Autodesk Fusion 360 part; units mm, degrees
(part 4 of 6)
  line L2387 (33.796111, 261.14375) -> (33.866667, 261.14375)
  line L2388 (10.442222, 231.61625) -> (10.089444, 231.475139)
  line L2389 (7.796389, 232.180694) -> (8.043333, 231.93375)
  line L2390 (28.998333, 231.651528) -> (29.068889, 231.722083)
  line L2391 (29.068889, 231.722083) -> (29.068889, 231.792639)
  line L2392 (28.292778, 227.347639) -> (28.222222, 227.312361)
  line L2393 (28.222222, 227.312361) -> (28.186944, 227.277083)
  line L2394 (28.186944, 227.277083) -> (28.151667, 227.17125)
  line L2395 (9.419167, 223.467083) -> (9.419167, 227.030139)
  line L2396 (16.086667, 223.220139) -> (16.016111, 223.149583)
  line L2397 (23.600833, 231.051805) -> (23.706667, 231.016528)
  line L2398 (23.495, 231.228194) -> (23.495, 231.157639)
  line L2399 (23.212778, 288.025417) -> (23.248056, 287.954861)
  line L2400 (23.248056, 287.954861) -> (23.212778, 287.81375)
  line L2401 (23.212778, 287.81375) -> (23.1775, 287.778472)
  line L2402 (5.961944, 223.184861) -> (6.067778, 223.114305)
  line L2403 (27.305, 252.88875) -> (27.340278, 252.641805)
  line L2404 (35.454167, 262.378472) -> (34.360556, 262.378472)
  line L2405 (41.521944, 265.377083) -> (41.768889, 265.341805)
  line L2406 (34.395833, 287.990139) -> (34.536944, 287.919583)
  line L2407 (35.806944, 289.648194) -> (35.806944, 289.507083)
  line L2408 (13.229167, 227.030139) -> (13.264444, 227.17125)
  line L2409 (36.83, 227.382917) -> (39.0525, 227.382917)
  line L2410 (43.991389, 288.836805) -> (43.991389, 287.390417)
  line L2411 (31.291389, 257.01625) -> (31.538333, 257.157361)
  line L2412 (31.538333, 257.157361) -> (31.785278, 257.369028)
  line L2413 (31.785278, 257.369028) -> (31.996944, 257.615972)
  line L2414 (31.996944, 257.615972) -> (32.138056, 257.898194)
  line L2415 (42.721389, 272.503194) -> (42.721389, 272.57375)
  line L2416 (42.721389, 272.57375) -> (42.686111, 272.644305)
  line L2417 (42.474444, 272.25625) -> (42.580278, 272.25625)
  line L2418 (8.396111, 226.85375) -> (8.501944, 226.85375)
  line L2419 (8.501944, 226.85375) -> (8.643056, 226.889028)
  line L2420 (8.643056, 226.889028) -> (8.678333, 226.924305)
  line L2421 (39.087778, 276.771805) -> (39.017222, 276.807083)
  line L2422 (39.193611, 276.277917) -> (39.228889, 276.419028)
  line L2423 (23.918333, 229.993472) -> (23.988889, 229.640694)
  line L2424 (17.78, 290.283194) -> (17.603611, 290.459583)
  line L2425 (13.440833, 223.114305) -> (13.335, 223.184861)
  line L2426 (14.781389, 280.722917) -> (14.499167, 280.687639)
  line L2427 (14.499167, 280.687639) -> (14.181667, 280.581805)
  line L2428 (14.181667, 280.581805) -> (13.899444, 280.440694)
  line L2429 (13.899444, 280.440694) -> (13.6525, 280.264305)
  line L2430 (39.299444, 265.659305) -> (39.405278, 265.624028)
  line L2431 (9.666111, 223.114305) -> (9.807222, 223.184861)
  line L2432 (9.807222, 223.184861) -> (9.877778, 223.220139)
  line L2433 (9.877778, 223.220139) -> (9.913056, 223.255417)
  line L2434 (26.387778, 253.20625) -> (26.916944, 253.20625)
  line L2435 (9.383889, 231.369305) -> (9.736667, 231.404583)
  line L2436 (15.769167, 223.114305) -> (13.581944, 223.114305)
  line L2437 (22.895278, 225.548472) -> (22.754167, 225.548472)
  line L2438 (23.106944, 224.172639) -> (23.106944, 225.195694)
  line L2439 (22.965833, 223.643472) -> (23.106944, 223.925694)
  line L2440 (23.106944, 223.925694) -> (23.106944, 224.172639)
  line L2441 (32.208611, 227.135972) -> (32.208611, 227.206528)
  line L2442 (32.208611, 227.206528) -> (32.138056, 227.277083)
  line L2443 (32.138056, 227.277083) -> (32.102778, 227.347639)
  line L2444 (40.181389, 240.329861) -> (40.287222, 240.400417)
  line L2445 (40.287222, 240.400417) -> (40.3225, 240.470972)
  line L2446 (40.3225, 240.470972) -> (40.357778, 240.541528)
  line L2447 (34.113611, 223.220139) -> (34.184167, 223.149583)
  line L2448 (34.184167, 223.149583) -> (34.325278, 223.114305)
  line L2449 (34.043056, 223.467083) -> (34.043056, 223.396528)
  line L2450 (31.185556, 291.094583) -> (31.256111, 291.165139)
  line L2451 (30.832778, 291.165139) -> (30.903333, 291.129861)
  line L2452 (35.806944, 285.873472) -> (35.771667, 285.661805)
  line L2453 (36.124444, 272.503194) -> (36.089167, 272.57375)
  line L2454 (36.089167, 272.57375) -> (36.089167, 272.644305)
  line L2455 (23.883056, 231.157639) -> (23.847778, 231.087083)
  line L2456 (23.847778, 231.087083) -> (23.777222, 231.051805)
  line L2457 (23.777222, 231.051805) -> (23.706667, 231.016528)
  line L2458 (42.545, 264.459861) -> (42.509722, 264.354028)
  line L2459 (38.064722, 245.692083) -> (38.029444, 245.58625)
  line L2460 (13.299722, 227.277083) -> (13.440833, 227.347639)
  line L2461 (38.029444, 245.58625) -> (38.029444, 245.515694)
  line L2462 (39.0525, 248.902361) -> (38.064722, 245.692083)
  line L2463 (39.264167, 249.07875) -> (39.193611, 249.07875)
  line L2464 (39.193611, 249.07875) -> (39.123056, 249.043472)
  line L2465 (30.938611, 291.059305) -> (31.079722, 291.059305)
  line L2466 (30.832778, 291.341528) -> (30.832778, 291.235694)
  line L2467 (30.832778, 291.235694) -> (30.832778, 291.165139)
  line L2468 (42.545, 262.202083) -> (42.545, 261.955139)
  line L2469 (42.2275, 263.542639) -> (41.733611, 263.542639)
  line L2470 (19.332222, 225.407361) -> (19.508611, 225.760139)
  line L2471 (36.053889, 272.326805) -> (36.089167, 272.397361)
  line L2472 (36.089167, 272.397361) -> (36.124444, 272.503194)
  line L2473 (39.264167, 276.524861) -> (39.264167, 276.665972)
  line L2474 (31.397222, 229.07625) -> (31.4325, 229.040972)
  line L2475 (38.770278, 276.665972) -> (38.876111, 276.736528)
  line L2476 (27.6225, 231.61625) -> (28.821944, 231.61625)
  line L2477 (27.6225, 230.769583) -> (27.6225, 231.61625)
  line L2478 (20.073056, 290.283194) -> (17.78, 290.283194)
  line L2479 (38.205833, 233.168472) -> (38.205833, 233.027361)
  line L2480 (38.205833, 233.027361) -> (38.276389, 232.921528)
  line L2481 (31.291389, 291.270972) -> (31.291389, 291.341528)
  line L2482 (6.067778, 223.114305) -> (6.173611, 223.114305)
  line L2483 (5.856111, 227.030139) -> (5.856111, 223.467083)
  line L2484 (38.523333, 249.537361) -> (38.488056, 249.502083)
  line L2485 (18.626667, 226.783194) -> (18.803056, 226.677361)
  line L2486 (34.29, 291.200417) -> (34.395833, 291.094583)
  line L2487 (34.360556, 262.378472) -> (34.925, 264.212917)
  line L2488 (34.713333, 275.325417) -> (35.277778, 273.490972)
  line L2489 (40.498889, 245.58625) -> (40.534167, 245.515694)
  line L2490 (40.534167, 245.515694) -> (40.498889, 245.445139)
  line L2491 (40.498889, 245.445139) -> (40.463611, 245.374583)
  line L2492 (40.463611, 245.374583) -> (40.393056, 245.304028)
  line L2493 (40.393056, 245.304028) -> (40.287222, 245.304028)
  line L2494 (40.287222, 245.304028) -> (40.216667, 245.304028)
  line L2495 (40.216667, 245.304028) -> (40.146111, 245.339305)
  line L2496 (40.146111, 245.339305) -> (40.075556, 245.409861)
  line L2497 (40.075556, 245.409861) -> (40.040278, 245.480417)
  line L2498 (40.040278, 245.480417) -> (39.899167, 245.939028)
  line L2499 (39.899167, 245.939028) -> (38.629167, 245.939028)
  line L2500 (38.629167, 245.939028) -> (38.488056, 245.445139)
  line L2501 (38.488056, 245.445139) -> (38.452778, 245.374583)
  line L2502 (38.452778, 245.374583) -> (38.4175, 245.339305)
  line L2503 (38.4175, 245.339305) -> (38.346944, 245.304028)
  line L2504 (38.346944, 245.304028) -> (38.276389, 245.304028)
  line L2505 (38.276389, 245.304028) -> (38.135278, 245.339305)
  line L2506 (38.135278, 245.339305) -> (38.064722, 245.409861)
  line L2507 (38.064722, 245.409861) -> (38.029444, 245.515694)
  line L2508 (38.029444, 245.515694) -> (38.029444, 245.58625)
  line L2509 (38.029444, 245.58625) -> (38.064722, 245.692083)
  line L2510 (38.064722, 245.692083) -> (39.0525, 248.902361)
  line L2511 (39.0525, 248.902361) -> (39.0525, 248.972917)
  line L2512 (39.0525, 248.972917) -> (39.123056, 249.043472)
  line L2513 (39.123056, 249.043472) -> (39.193611, 249.07875)
  line L2514 (39.193611, 249.07875) -> (39.264167, 249.07875)
  line L2515 (39.264167, 249.07875) -> (39.334722, 249.07875)
  line L2516 (39.334722, 249.07875) -> (39.405278, 249.043472)
  line L2517 (39.405278, 249.043472) -> (39.475833, 248.972917)
  line L2518 (39.475833, 248.972917) -> (39.511111, 248.867083)
  line L2519 (39.511111, 248.867083) -> (40.498889, 245.656805)
  line L2520 (40.498889, 245.656805) -> (40.498889, 245.58625)
  line L2521 (27.163889, 223.114305) -> (27.657778, 223.220139)
  line L2522 (27.657778, 223.220139) -> (28.116389, 223.431805)
  line L2523 (28.116389, 223.431805) -> (28.363333, 223.714028)
  line L2524 (40.569444, 261.743472) -> (40.781111, 261.46125)
  line L2525 (40.781111, 261.46125) -> (41.028056, 261.249583)
  line L2526 (41.028056, 261.249583) -> (41.275, 261.179028)
  line L2527 (8.184444, 225.513194) -> (8.149167, 225.372083)
  line L2528 (8.149167, 225.372083) -> (8.113889, 225.336805)
  line L2529 (24.4475, 253.559028) -> (24.412222, 253.594305)
  line L2530 (24.412222, 253.594305) -> (24.341667, 253.594305)
  line L2531 (25.4, 250.630972) -> (24.553333, 253.417917)
  line L2532 (23.8125, 285.90875) -> (23.8125, 285.838194)
  line L2533 (23.106944, 224.172639) -> (23.106944, 223.925694)
  line L2534 (23.106944, 223.925694) -> (22.965833, 223.643472)
  line L2535 (23.248056, 229.111528) -> (23.389167, 229.182083)
  line L2536 (23.389167, 229.182083) -> (23.530278, 229.358472)
  line L2537 (23.530278, 229.358472) -> (23.565556, 229.640694)
  line L2538 (39.017222, 241.599861) -> (38.911389, 241.635139)
  line L2539 (38.911389, 241.635139) -> (38.770278, 241.77625)
  line L2540 (30.903333, 291.129861) -> (30.938611, 291.059305)
  line L2541 (8.149167, 225.58375) -> (8.113889, 225.689583)
  line L2542 (18.273889, 226.85375) -> (18.485556, 226.85375)
  line L2543 (38.946667, 276.807083) -> (38.876111, 276.736528)
  line L2544 (38.876111, 276.736528) -> (38.770278, 276.665972)
  line L2545 (42.2275, 272.432639) -> (42.262778, 272.362083)
  line L2546 (34.572222, 223.36125) -> (34.572222, 223.431805)
  line L2547 (34.325278, 223.114305) -> (34.466389, 223.149583)
  line L2548 (34.466389, 223.149583) -> (34.536944, 223.255417)
  line L2549 (29.845, 225.26625) -> (31.291389, 225.26625)
  line L2550 (29.845, 223.643472) -> (29.845, 225.26625)
  line L2551 (31.891111, 223.643472) -> (29.845, 223.643472)
  line L2552 (22.613056, 231.369305) -> (22.718889, 231.545694)
  line L2553 (22.648333, 230.804861) -> (22.577778, 230.98125)
  line L2554 (22.930556, 226.889028) -> (23.036389, 226.747917)
  line L2555 (11.006667, 225.372083) -> (12.100278, 227.206528)
  line L2556 (25.011944, 290.283194) -> (23.459722, 290.283194)
  line L2557 (25.153056, 229.675972) -> (25.576389, 231.087083)
  line L2558 (30.973889, 256.945694) -> (31.291389, 257.01625)
  line L2559 (28.433889, 289.295417) -> (28.222222, 289.330694)
  line L2560 (21.484167, 290.283194) -> (26.3525, 295.151528)
  line L2561 (27.199167, 285.555972) -> (27.305, 285.59125)
  line L2562 (21.201944, 223.99625) -> (21.484167, 223.749305)
  line L2563 (42.545, 263.189861) -> (42.545, 263.36625)
  line L2564 (42.545, 263.36625) -> (42.474444, 263.507361)
  line L2565 (40.040278, 232.88625) -> (40.287222, 232.921528)
  line L2566 (40.287222, 232.921528) -> (40.3225, 232.956805)
  line L2567 (32.138056, 257.898194) -> (32.208611, 258.180417)
  line L2568 (29.986111, 229.111528) -> (31.220833, 229.111528)
  line L2569 (28.575, 224.066805) -> (28.645556, 224.419583)
  line L2570 (28.645556, 224.419583) -> (28.680833, 224.701805)
  line L2571 (32.208611, 279.452917) -> (32.138056, 279.735139)
  line L2572 (32.138056, 279.735139) -> (31.996944, 280.017361)
  line L2573 (31.996944, 280.017361) -> (31.785278, 280.264305)
  line L2574 (31.785278, 280.264305) -> (31.538333, 280.440694)
  line L2575 (8.713611, 223.537639) -> (8.748889, 223.467083)
  line L2576 (8.748889, 223.467083) -> (8.748889, 223.396528)
  line L2577 (11.183056, 224.666528) -> (11.288889, 224.807639)
  line L2578 (8.113889, 225.336805) -> (8.078611, 225.301528)
  line L2579 (8.078611, 225.301528) -> (7.831667, 225.26625)
  line L2580 (32.208611, 258.180417) -> (32.243889, 258.497917)
  line L2581 (14.781389, 256.910417) -> (30.656389, 256.910417)
  line L2582 (13.193889, 258.497917) -> (13.229167, 258.180417)
  line L2583 (13.229167, 258.180417) -> (13.335, 257.898194)
  line L2584 (22.295556, 231.686805) -> (22.189722, 231.404583)
  line L2585 (22.189722, 231.404583) -> (22.154444, 231.157639)
  line L2586 (21.096111, 227.100694) -> (20.672778, 226.677361)
  line L2587 (20.672778, 226.677361) -> (20.390556, 226.148194)
  line L2588 (29.739167, 285.59125) -> (29.809722, 285.697083)
  line L2589 (29.315833, 285.732361) -> (29.351111, 285.661805)
  line L2590 (6.561667, 295.821805) -> (6.279444, 295.574861)
  line L2591 (6.279444, 295.574861) -> (6.420556, 295.821805)
  line L2592 (31.326667, 231.61625) -> (31.220833, 231.61625)
  line L2593 (29.315833, 285.90875) -> (29.315833, 285.838194)
  line L2594 (24.906111, 285.626528) -> (25.011944, 285.767639)
  line L2595 (28.433889, 289.295417) -> (29.315833, 289.295417)
  line L2596 (28.116389, 289.471805) -> (28.151667, 289.40125)
  line L2597 (25.153056, 289.754028) -> (25.0825, 289.789305)
  line L2598 (25.0825, 289.789305) -> (25.011944, 289.824583)
  line L2599 (31.220833, 231.61625) -> (29.986111, 231.61625)
  line L2600 (29.986111, 231.61625) -> (29.986111, 230.769583)
  line L2601 (29.351111, 285.661805) -> (29.421667, 285.59125)
  line L2602 (29.421667, 285.59125) -> (29.562778, 285.555972)
  line L2603 (29.986111, 230.769583) -> (30.868056, 230.769583)
  line L2604 (42.580278, 264.565694) -> (42.545, 264.459861)
  line L2605 (42.015833, 262.131528) -> (42.051111, 262.343194)
  line L2606 (22.436667, 229.817083) -> (22.471944, 229.71125)
  line L2607 (22.471944, 229.71125) -> (22.507222, 229.605417)
  line L2608 (22.507222, 229.605417) -> (22.507222, 229.429028)
  line L2609 (30.868056, 230.769583) -> (31.044444, 230.734305)
  line L2610 (31.044444, 230.734305) -> (31.079722, 230.699028)
  line L2611 (31.079722, 230.699028) -> (31.115, 230.628472)
  line L2612 (31.115, 230.628472) -> (31.115, 230.557917)
  line L2613 (24.553333, 285.626528) -> (24.659167, 285.59125)
  line L2614 (24.659167, 285.59125) -> (24.729722, 285.555972)
  line L2615 (30.973889, 289.365972) -> (31.009167, 289.436528)
  line L2616 (24.482778, 285.697083) -> (24.553333, 285.626528)
  line L2617 (27.446111, 285.944028) -> (27.375556, 286.014583)
  line L2618 (27.305, 285.59125) -> (27.410833, 285.661805)
  line L2619 (8.995833, 231.439861) -> (8.643056, 231.545694)
  line L2620 (30.691667, 289.295417) -> (30.938611, 289.330694)
  line L2621 (30.938611, 289.330694) -> (30.973889, 289.365972)
  line L2622 (31.009167, 289.436528) -> (31.044444, 289.542361)
  line L2623 (29.845, 289.295417) -> (30.691667, 289.295417)
  line L2624 (34.078333, 286.579028) -> (34.113611, 286.790694)
  line L2625 (34.113611, 286.790694) -> (34.113611, 287.460972)
  line L2626 (9.383889, 231.369305) -> (8.995833, 231.439861)
  line L2627 (9.807222, 227.312361) -> (9.913056, 227.17125)
  line L2628 (18.203333, 289.260139) -> (18.0975, 289.648194)
  line L2629 (18.0975, 289.648194) -> (17.956389, 289.965694)
  line L2630 (24.870833, 228.794028) -> (24.906111, 228.829305)
  line L2631 (24.482778, 228.899861) -> (24.518056, 228.794028)
  line L2632 (23.212778, 288.025417) -> (23.1775, 288.13125)
  line L2633 (23.706667, 289.330694) -> (23.741944, 289.365972)
  line L2634 (23.741944, 289.365972) -> (23.777222, 289.436528)
  line L2635 (23.8125, 285.838194) -> (23.8125, 285.697083)
  line L2636 (23.8125, 285.697083) -> (23.777222, 285.626528)
  line L2637 (23.777222, 285.626528) -> (23.706667, 285.59125)
  line L2638 (17.956389, 289.965694) -> (17.78, 290.283194)
  line L2639 (16.051389, 286.296805) -> (16.051389, 286.825972)
  line L2640 (25.646944, 287.884305) -> (24.553333, 286.049861)
  line L2641 (29.315833, 285.838194) -> (29.315833, 285.90875)
  line L2642 (38.770278, 246.397639) -> (39.264167, 248.020417)
  line L2643 (8.643056, 231.545694) -> (8.325556, 231.686805)
  line L2644 (28.151667, 289.40125) -> (28.116389, 289.471805)
  line L2645 (8.325556, 231.686805) -> (8.043333, 231.93375)
  line L2646 (26.458333, 228.723472) -> (26.564167, 228.723472)
  line L2647 (26.564167, 228.723472) -> (26.634722, 228.75875)
  line L2648 (29.5275, 293.599305) -> (29.598056, 293.564028)
  line L2649 (27.410833, 285.661805) -> (27.446111, 285.732361)
  line L2650 (29.845, 285.873472) -> (29.845, 289.295417)
  line L2651 (29.845, 285.802917) -> (29.845, 285.873472)
  line L2652 (31.115, 230.487361) -> (31.079722, 230.416805)
  line L2653 (39.334722, 284.885694) -> (35.136667, 284.885694)
  line L2654 (31.115, 230.557917) -> (31.115, 230.487361)
  line L2655 (29.809722, 285.697083) -> (29.845, 285.802917)
  line L2656 (12.453056, 227.347639) -> (12.523611, 227.312361)
  line L2657 (25.011944, 290.283194) -> (26.3525, 290.283194)
  line L2658 (17.78, 290.283194) -> (20.073056, 290.283194)
  line L2659 (16.051389, 286.825972) -> (16.439444, 286.86125)
  line L2660 (16.439444, 286.86125) -> (16.792222, 286.931805)
  line L2661 (17.427222, 287.284583) -> (17.674167, 287.566805)
  line L2662 (17.674167, 287.566805) -> (17.921111, 287.849028)
  line L2663 (28.151667, 289.683472) -> (28.186944, 289.71875)
  line L2664 (17.921111, 287.849028) -> (18.062222, 288.201805)
  line L2665 (18.062222, 288.201805) -> (18.168056, 288.554583)
  line L2666 (18.168056, 288.554583) -> (18.203333, 288.907361)
  line L2667 (18.203333, 288.907361) -> (18.203333, 289.260139)
  line L2668 (39.722778, 231.863194) -> (39.793333, 231.686805)
  line L2669 (39.793333, 231.686805) -> (39.828611, 231.404583)
  line L2670 (23.988889, 229.640694) -> (23.953611, 229.323194)
  line L2671 (42.580278, 272.25625) -> (42.686111, 272.326805)
  line L2672 (42.686111, 272.326805) -> (42.721389, 272.397361)
  line L2673 (34.219444, 294.234305) -> (34.254722, 294.057917)
  line L2674 (39.828611, 231.404583) -> (39.793333, 231.087083)
  line L2675 (35.630556, 261.849305) -> (35.806944, 261.320139)
  line L2676 (34.219444, 261.849305) -> (35.630556, 261.849305)
  line L2677 (9.489722, 223.184861) -> (9.454444, 223.220139)
  line L2678 (28.116389, 289.577639) -> (28.151667, 289.683472)
  line L2679 (34.007778, 293.52875) -> (33.866667, 293.422917)
  line L2680 (33.831389, 294.728194) -> (34.043056, 294.587083)
  line L2681 (33.655, 293.352361) -> (33.443333, 293.352361)
  line L2682 (34.254722, 294.057917) -> (34.219444, 293.84625)
  line L2683 (39.793333, 231.087083) -> (39.652222, 230.910694)
  line L2684 (39.37, 232.039583) -> (39.511111, 232.039583)
  line L2685 (9.666111, 223.114305) -> (9.525, 223.149583)
  line L2686 (27.128611, 253.135694) -> (27.234444, 253.029861)
  line L2687 (22.577778, 246.820972) -> (22.048611, 246.397639)
  line L2688 (22.048611, 246.397639) -> (21.59, 245.939028)
  line L2689 (21.59, 245.939028) -> (21.166667, 245.445139)
  line L2690 (21.166667, 245.445139) -> (20.813889, 244.880694)
  line L2691 (19.05, 226.148194) -> (19.014722, 225.936528)
  line L2692 (19.014722, 225.936528) -> (18.908889, 225.724861)
  line L2693 (26.67, 228.899861) -> (26.67, 228.970417)
  line L2694 (26.67, 228.970417) -> (26.634722, 229.040972)
  line L2695 (28.116389, 289.471805) -> (28.116389, 289.577639)
  line L2696 (39.475833, 230.769583) -> (39.334722, 230.769583)
  line L2697 (39.581667, 231.969028) -> (39.722778, 231.863194)
  line L2698 (26.67, 228.899861) -> (26.67, 228.829305)
  line L2699 (26.67, 228.829305) -> (26.634722, 228.75875)
  line L2700 (26.634722, 228.75875) -> (26.564167, 228.723472)
  line L2701 (26.564167, 228.723472) -> (26.458333, 228.723472)
  line L2702 (26.458333, 228.723472) -> (26.387778, 228.723472)
  line L2703 (26.387778, 228.723472) -> (26.3525, 228.723472)
  line L2704 (26.3525, 228.723472) -> (26.281944, 228.794028)
  line L2705 (26.281944, 228.794028) -> (26.246667, 228.864583)
  line L2706 (26.246667, 228.864583) -> (26.140833, 229.252639)
  line L2707 (26.140833, 229.252639) -> (25.011944, 229.252639)
  line L2708 (25.011944, 229.252639) -> (24.906111, 228.829305)
  line L2709 (24.906111, 228.829305) -> (24.870833, 228.794028)
  line L2710 (24.870833, 228.794028) -> (24.835556, 228.75875)
  line L2711 (24.835556, 228.75875) -> (24.765, 228.723472)
  line L2712 (24.765, 228.723472) -> (24.694444, 228.723472)
  line L2713 (24.694444, 228.723472) -> (24.588611, 228.75875)
  line L2714 (24.588611, 228.75875) -> (24.518056, 228.794028)
  line L2715 (24.518056, 228.794028) -> (24.482778, 228.899861)
  line L2716 (24.482778, 228.899861) -> (24.518056, 228.970417)
  line L2717 (24.518056, 228.970417) -> (24.518056, 229.07625)
  line L2718 (24.518056, 229.07625) -> (25.364722, 231.863194)
  line L2719 (25.364722, 231.863194) -> (25.4, 231.93375)
  line L2720 (25.4, 231.93375) -> (25.435278, 231.969028)
  line L2721 (25.435278, 231.969028) -> (25.505833, 232.004305)
  line L2722 (25.505833, 232.004305) -> (25.576389, 232.004305)
  line L2723 (25.576389, 232.004305) -> (25.646944, 232.004305)
  line L2724 (25.646944, 232.004305) -> (25.7175, 231.969028)
  line L2725 (25.7175, 231.969028) -> (25.752778, 231.898472)
  line L2726 (25.752778, 231.898472) -> (25.788056, 231.827917)
  line L2727 (25.788056, 231.827917) -> (26.634722, 229.040972)
  line L2728 (26.634722, 229.040972) -> (26.67, 228.970417)
  line L2729 (26.67, 228.970417) -> (26.67, 228.899861)
  line L2730 (39.511111, 232.039583) -> (39.581667, 231.969028)
  line L2731 (38.735, 232.039583) -> (39.37, 232.039583)
  line L2732 (39.652222, 230.910694) -> (39.581667, 230.840139)
  line L2733 (39.581667, 230.840139) -> (39.475833, 230.769583)
  line L2734 (38.735, 230.769583) -> (38.735, 232.039583)
  line L2735 (39.334722, 230.769583) -> (38.735, 230.769583)
  line L2736 (27.199167, 284.885694) -> (27.375556, 284.885694)
  line L2737 (6.279444, 295.574861) -> (6.561667, 295.821805)
  line L2738 (6.279444, 295.574861) -> (5.150556, 292.999583)
  line L2739 (19.861389, 242.446528) -> (19.790833, 241.811528)
  line L2740 (19.790833, 241.811528) -> (19.755556, 241.14125)
  line L2741 (26.3525, 295.151528) -> (26.3525, 290.283194)
  line L2742 (6.420556, 295.821805) -> (6.279444, 295.574861)
  line L2743 (6.561667, 295.821805) -> (6.420556, 295.821805)
  line L2744 (20.214167, 243.716528) -> (20.0025, 243.116805)
  line L2745 (20.0025, 243.116805) -> (19.861389, 242.446528)
  line L2746 (31.044444, 230.416805) -> (30.938611, 230.381528)
  line L2747 (20.813889, 244.880694) -> (20.496389, 244.31625)
  line L2748 (20.496389, 244.31625) -> (20.214167, 243.716528)
  line L2749 (33.513889, 294.763472) -> (33.690278, 294.763472)
  line L2750 (33.690278, 294.763472) -> (33.831389, 294.728194)
  line L2751 (33.443333, 293.352361) -> (32.526111, 293.352361)
  line L2752 (33.866667, 293.422917) -> (33.655, 293.352361)
  line L2753 (30.233056, 250.313472) -> (30.127222, 250.313472)
  line L2754 (32.526111, 294.763472) -> (33.513889, 294.763472)
  line L2755 (32.526111, 293.352361) -> (32.526111, 294.763472)
  line L2756 (12.558889, 227.206528) -> (12.594167, 227.100694)
  line L2757 (7.972778, 295.821805) -> (5.150556, 292.999583)
  line L2758 (7.972778, 295.821805) -> (6.561667, 295.821805)
  line L2759 (19.261667, 295.821805) -> (14.322778, 295.821805)
  line L2760 (1.446389, 282.945417) -> (1.446389, 281.745972)
  line L2761 (28.398611, 253.594305) -> (28.469167, 253.594305)
  line L2762 (5.185833, 281.745972) -> (19.261667, 295.821805)
  line L2763 (1.446389, 284.391805) -> (12.911667, 295.821805)
  line L2764 (27.022778, 253.170972) -> (27.128611, 253.135694)
  line L2765 (25.999722, 229.675972) -> (25.153056, 229.675972)
  line L2766 (25.576389, 231.087083) -> (25.999722, 229.675972)
  line L2767 (39.698083, 284.522333) -> (43.991389, 288.836805)
  line L2768 (11.535833, 281.745972) -> (16.051389, 286.296805)
  line L2769 (27.798889, 293.705139) -> (29.245278, 293.705139)
  line L2770 (23.8125, 231.61625) -> (23.847778, 231.439861)
  line L2771 (23.847778, 231.439861) -> (23.883056, 231.228194)
  line L2772 (23.883056, 231.228194) -> (23.883056, 231.157639)
  line L2773 (16.086667, 284.885694) -> (16.051389, 284.885694)
  line L2774 (21.025556, 284.885694) -> (16.086667, 284.885694)
  line L2775 (28.786667, 284.885694) -> (25.646944, 281.745972)
  line L2776 (22.436667, 284.885694) -> (19.296944, 281.745972)
  line L2777 (41.416111, 263.401528) -> (41.451389, 263.472083)
  line L2778 (25.435278, 250.560417) -> (25.435278, 250.489861)
  line L2779 (25.435278, 250.489861) -> (25.4, 250.419305)
  line L2780 (25.4, 250.419305) -> (25.364722, 250.34875)
  line L2781 (25.364722, 250.34875) -> (25.294167, 250.313472)
  line L2782 (25.294167, 250.313472) -> (25.223611, 250.313472)
  line L2783 (25.223611, 250.313472) -> (25.153056, 250.313472)
  line L2784 (25.153056, 250.313472) -> (25.117778, 250.313472)
  line L2785 (25.117778, 250.313472) -> (25.047222, 250.384028)
  line L2786 (25.047222, 250.384028) -> (25.011944, 250.454583)
  line L2787 (25.011944, 250.454583) -> (24.906111, 250.842639)
  line L2788 (24.906111, 250.842639) -> (23.777222, 250.842639)
  line L2789 (23.777222, 250.842639) -> (23.671389, 250.419305)
  line L2790 (23.671389, 250.419305) -> (23.636111, 250.384028)
  line L2791 (23.636111, 250.384028) -> (23.600833, 250.34875)
  line L2792 (23.600833, 250.34875) -> (23.530278, 250.313472)
  line L2793 (23.530278, 250.313472) -> (23.459722, 250.313472)
  line L2794 (23.459722, 250.313472) -> (23.318611, 250.34875)
  line L2795 (23.318611, 250.34875) -> (23.283333, 250.384028)
  line L2796 (23.283333, 250.384028) -> (23.248056, 250.489861)
  line L2797 (23.248056, 250.489861) -> (23.248056, 250.560417)
  line L2798 (23.248056, 250.560417) -> (23.283333, 250.66625)
  line L2799 (23.283333, 250.66625) -> (24.13, 253.453194)
  line L2800 (24.13, 253.453194) -> (24.165278, 253.52375)
  line L2801 (24.165278, 253.52375) -> (24.200556, 253.559028)
  line L2802 (24.200556, 253.559028) -> (24.271111, 253.594305)
  line L2803 (24.271111, 253.594305) -> (24.341667, 253.594305)
  line L2804 (24.341667, 253.594305) -> (24.412222, 253.594305)
  line L2805 (24.412222, 253.594305) -> (24.4475, 253.559028)
  line L2806 (24.4475, 253.559028) -> (24.518056, 253.488472)
  line L2807 (24.518056, 253.488472) -> (24.553333, 253.417917)
  line L2808 (24.553333, 253.417917) -> (25.4, 250.630972)
  line L2809 (25.4, 250.630972) -> (25.435278, 250.560417)
  line L2810 (23.706667, 231.016528) -> (23.777222, 231.051805)
  line L2811 (23.777222, 231.051805) -> (23.847778, 231.087083)
  line L2812 (40.040278, 249.537361) -> (40.075556, 249.502083)
  line L2813 (40.075556, 249.502083) -> (40.146111, 249.466805)
  line L2814 (40.146111, 249.466805) -> (40.216667, 249.431528)
  line L2815 (32.843611, 227.135972) -> (32.878889, 227.241805)
  line L2816 (8.678333, 226.924305) -> (8.643056, 226.889028)
  line L2817 (8.643056, 226.889028) -> (8.501944, 226.85375)
  line L2818 (34.925, 264.212917) -> (35.454167, 262.378472)
  line L2819 (35.454167, 262.378472) -> (34.360556, 262.378472)
  line L2820 (13.476111, 257.615972) -> (13.6525, 257.369028)
  line L2821 (13.6525, 257.369028) -> (13.899444, 257.157361)
  line L2822 (13.899444, 257.157361) -> (14.181667, 257.01625)
  line L2823 (14.181667, 257.01625) -> (14.499167, 256.945694)
  line L2824 (23.847778, 231.087083) -> (23.883056, 231.157639)
  line L2825 (23.883056, 231.157639) -> (23.883056, 231.228194)
  line L2826 (38.205833, 236.449305) -> (38.205833, 236.343472)
  line L2827 (40.075556, 236.660972) -> (38.523333, 236.660972)
  line L2828 (40.675278, 263.260417) -> (40.675278, 262.907639)
  line L2829 (22.648333, 230.34625) -> (22.471944, 230.416805)
  line L2830 (22.471944, 230.416805) -> (22.330833, 230.557917)
  line L2831 (22.330833, 230.557917) -> (22.260278, 230.699028)
  line L2832 (38.135278, 253.100417) -> (38.1, 252.924028)
  line L2833 (29.315833, 285.90875) -> (29.315833, 289.295417)
  line L2834 (13.581944, 227.382917) -> (15.804444, 227.382917)
  line L2835 (27.693056, 250.66625) -> (27.693056, 250.701528)
  line L2836 (27.763611, 250.525139) -> (27.763611, 250.560417)
  line L2837 (25.435278, 218.034306) -> (30.374167, 218.034306)
  line L2838 (43.991389, 218.986806) -> (43.991389, 218.034306)
  line L2839 (43.991389, 218.034306) -> (43.074167, 218.034306)
  line L2840 (38.4175, 245.339305) -> (38.452778, 245.374583)
  line L2841 (23.530278, 228.794028) -> (23.142222, 228.723472)
  line L2842 (31.467778, 231.827917) -> (31.467778, 231.863194)
  line L2843 (31.467778, 231.863194) -> (31.4325, 231.93375)
  line L2844 (31.4325, 231.93375) -> (31.361944, 231.969028)
  line L2845 (43.074167, 218.034306) -> (43.991389, 218.986806)
  line L2846 (43.991389, 222.549861) -> (43.991389, 218.986806)
  line L2847 (43.991389, 218.986806) -> (43.074167, 218.034306)
  line L2848 (43.074167, 218.034306) -> (38.135278, 218.034306)
  line L2849 (36.83, 272.57375) -> (36.865278, 272.679583)
  line L2850 (40.075556, 249.502083) -> (40.040278, 249.537361)
  line L2851 (37.323889, 272.397361) -> (37.218056, 272.291528)
  line L2852 (40.851667, 264.212917) -> (40.710556, 263.754305)
  line L2853 (41.133889, 264.63625) -> (40.992778, 264.424583)
  line L2854 (23.142222, 232.004305) -> (22.895278, 232.004305)
  line L2855 (23.1775, 232.004305) -> (23.142222, 232.004305)
  line L2856 (22.895278, 232.004305) -> (23.142222, 232.004305)
  line L2857 (23.142222, 232.004305) -> (23.1775, 232.004305)
  line L2858 (23.1775, 232.004305) -> (23.353889, 232.004305)
  line L2859 (40.393056, 262.060972) -> (40.287222, 262.378472)
  line L2860 (41.557222, 264.847917) -> (41.310278, 264.777361)
  line L2861 (30.868056, 295.186805) -> (30.832778, 295.080972)
  line L2862 (33.408056, 287.49625) -> (33.3375, 287.566805)
  line L2863 (33.3375, 287.566805) -> (33.302222, 287.707917)
  line L2864 (7.831667, 225.26625) -> (6.385278, 225.26625)
  line L2865 (6.385278, 225.26625) -> (6.385278, 223.643472)
  line L2866 (41.521944, 261.14375) -> (41.275, 261.179028)
  line L2867 (42.2275, 264.248194) -> (42.156944, 264.283472)
  line L2868 (20.990278, 224.31375) -> (21.201944, 223.99625)
  line L2869 (34.713333, 275.325417) -> (35.277778, 273.490972)
  line L2870 (41.451389, 263.472083) -> (41.521944, 263.507361)
  line L2871 (38.946667, 243.469583) -> (39.087778, 243.434305)
  line L2872 (40.393056, 245.304028) -> (40.463611, 245.374583)
  line L2873 (35.842222, 272.25625) -> (35.948056, 272.25625)
  line L2874 (35.948056, 272.25625) -> (36.053889, 272.326805)
  line L2875 (42.403889, 272.25625) -> (42.474444, 272.25625)
  line L2876 (42.051111, 272.961805) -> (42.2275, 272.432639)
  line L2877 (43.991389, 287.390417) -> (38.346944, 281.745972)
  line L2878 (33.443333, 286.085139) -> (33.196389, 286.120417)
  line L2879 (33.196389, 286.120417) -> (32.984722, 286.190972)
  line L2880 (31.4325, 229.040972) -> (31.467778, 228.970417)
  line L2881 (39.228889, 276.419028) -> (39.264167, 276.524861)
  line L2882 (37.323889, 272.397361) -> (39.193611, 276.277917)
  line L2883 (37.076944, 272.25625) -> (37.1475, 272.25625)
  line L2884 (39.017222, 276.807083) -> (39.087778, 276.771805)
  line L2885 (42.086389, 261.320139) -> (41.839444, 261.179028)
  line L2886 (23.706667, 231.016528) -> (23.600833, 231.051805)
  line L2887 (23.600833, 231.051805) -> (23.565556, 231.051805)
  line L2888 (23.565556, 231.051805) -> (23.530278, 231.122361)
  line L2889 (17.391944, 290.635972) -> (17.215556, 290.812361)
  line L2890 (36.865278, 272.714861) -> (38.770278, 276.665972)
  line L2891 (41.839444, 261.179028) -> (41.521944, 261.14375)
  line L2892 (40.781111, 262.590139) -> (40.922222, 262.166805)
  line L2893 (38.770278, 276.665972) -> (36.865278, 272.714861)
  line L2894 (39.017222, 276.807083) -> (38.946667, 276.807083)
  line L2895 (41.310278, 264.777361) -> (41.133889, 264.63625)
  line L2896 (27.199167, 228.970417) -> (27.199167, 231.722083)
  line L2897 (40.463611, 249.71375) -> (40.463611, 249.607917)
  line L2898 (32.173333, 226.994861) -> (32.208611, 227.100694)
  line L2899 (29.845, 226.85375) -> (31.855833, 226.85375)
  line L2900 (29.845, 225.760139) -> (29.845, 226.85375)
  line L2901 (22.895278, 232.004305) -> (22.5425, 231.898472)
  line L2902 (22.5425, 231.898472) -> (22.295556, 231.686805)
  line L2903 (10.089444, 231.475139) -> (9.736667, 231.404583)
  line L2904 (40.992778, 264.424583) -> (40.851667, 264.212917)
  line L2905 (33.549167, 287.990139) -> (33.655, 287.990139)
  line L2906 (31.079722, 291.059305) -> (30.938611, 291.059305)
  line L2907 (34.572222, 288.801528) -> (34.501667, 288.730972)
  line L2908 (34.501667, 288.730972) -> (34.360556, 288.695694)
  line L2909 (29.315833, 289.295417) -> (28.433889, 289.295417)
  line L2910 (33.866667, 261.14375) -> (33.9725, 261.179028)
  line L2911 (33.9725, 261.179028) -> (34.007778, 261.214305)
  line L2912 (34.007778, 261.214305) -> (34.043056, 261.284861)
  line L2913 (40.922222, 262.166805) -> (41.169167, 261.814028)
  line L2914 (9.454444, 227.241805) -> (9.489722, 227.312361)
  line L2915 (42.439167, 261.637639) -> (42.262778, 261.46125)
  line L2916 (34.325278, 223.114305) -> (34.184167, 223.149583)
  line L2917 (38.241111, 249.466805) -> (38.170556, 249.502083)
  line L2918 (31.855833, 222.549861) -> (34.325278, 222.549861)
  line L2919 (34.325278, 222.549861) -> (34.854444, 222.549861)
  line L2920 (38.664444, 233.344861) -> (38.664444, 234.755972)
  line L2921 (40.075556, 233.344861) -> (38.664444, 233.344861)
  line L2922 (40.357778, 233.097917) -> (40.357778, 233.168472)
  line L2923 (40.357778, 233.168472) -> (40.3225, 233.239028)
  line L2924 (17.603611, 290.459583) -> (17.391944, 290.635972)
  line L2925 (34.642778, 288.977917) -> (34.6075, 288.907361)
  line L2926 (34.6075, 288.907361) -> (34.572222, 288.801528)
  line L2927 (31.150278, 295.292639) -> (31.079722, 295.292639)
  line L2928 (31.291389, 291.341528) -> (31.291389, 295.010417)
  line L2929 (31.256111, 291.165139) -> (31.291389, 291.270972)
  line L2930 (7.796389, 232.180694) -> (7.584722, 232.498194)
  line L2931 (29.315833, 227.17125) -> (29.315833, 227.030139)
  line L2932 (31.891111, 227.382917) -> (29.668611, 227.382917)
  line L2933 (32.208611, 227.100694) -> (32.208611, 227.135972)
  line L2934 (29.668611, 223.114305) -> (31.855833, 223.114305)
  line L2935 (29.315833, 223.467083) -> (29.351111, 223.325972)
  line L2936 (29.351111, 223.325972) -> (29.421667, 223.184861)
  line L2937 (29.5275, 223.114305) -> (29.668611, 223.114305)
  line L2938 (29.315833, 227.030139) -> (29.315833, 223.467083)
  line L2939 (29.668611, 227.382917) -> (29.5275, 227.347639)
  line L2940 (42.262778, 261.46125) -> (42.086389, 261.320139)
  line L2941 (23.530278, 231.122361) -> (23.495, 231.157639)
  line L2942 (23.495, 231.157639) -> (23.495, 231.228194)
  line L2943 (23.495, 231.228194) -> (23.389167, 231.475139)
  line L2944 (38.346944, 281.745972) -> (36.935833, 281.745972)
  line L2945 (37.1475, 272.25625) -> (37.218056, 272.291528)
  line L2946 (37.218056, 272.291528) -> (37.323889, 272.397361)
  line L2947 (40.3225, 240.647361) -> (40.357778, 240.541528)
  line L2948 (32.7025, 286.437917) -> (32.490833, 286.755417)
  line L2949 (32.490833, 286.755417) -> (32.349722, 287.108194)
  line L2950 (33.231667, 227.382917) -> (35.454167, 227.382917)
  line L2951 (41.028056, 261.249583) -> (40.781111, 261.46125)
  line L2952 (29.5275, 227.347639) -> (29.386389, 227.277083)
  line L2953 (29.386389, 227.277083) -> (29.315833, 227.17125)
  line L2954 (32.984722, 286.190972) -> (32.7025, 286.437917)
  line L2955 (23.248056, 250.489861) -> (23.283333, 250.384028)
  line L2956 (20.849167, 224.666528) -> (20.990278, 224.31375)
  line L2957 (24.518056, 228.794028) -> (24.588611, 228.75875)
  line L2958 (24.588611, 228.75875) -> (24.694444, 228.723472)
  line L2959 (27.058056, 285.59125) -> (27.128611, 285.59125)
  line L2960 (27.128611, 285.59125) -> (27.199167, 285.555972)
  line L2961 (39.405278, 241.14125) -> (39.6875, 241.211805)
  line L2962 (31.009167, 289.683472) -> (30.938611, 289.754028)
  line L2963 (30.938611, 289.754028) -> (30.726944, 289.824583)
  line L2964 (8.678333, 227.277083) -> (8.713611, 227.206528)
  line L2965 (8.713611, 227.206528) -> (8.748889, 227.100694)
  line L2966 (34.043056, 223.290694) -> (34.043056, 223.396528)
  line L2967 (23.530278, 250.313472) -> (23.600833, 250.34875)
  line L2968 (23.600833, 250.34875) -> (23.636111, 250.384028)
  line L2969 (23.636111, 250.384028) -> (23.671389, 250.419305)
  line L2970 (19.508611, 223.572917) -> (19.473333, 223.608194)
  line L2971 (19.579167, 223.396528) -> (19.543889, 223.502361)
  line L2972 (19.543889, 223.502361) -> (19.508611, 223.572917)
  line L2973 (19.296944, 223.149583) -> (19.438056, 223.184861)
  line L2974 (34.995556, 276.242639) -> (34.925, 276.348472)
  line L2975 (34.925, 276.348472) -> (34.889722, 276.454305)
  line L2976 (20.778611, 224.94875) -> (20.849167, 224.666528)
  line L2977 (38.276389, 241.740972) -> (38.488056, 241.388194)
  line L2978 (38.488056, 241.388194) -> (38.770278, 241.211805)
  line L2979 (22.189722, 231.404583) -> (22.295556, 231.686805)
  line L2980 (22.295556, 231.686805) -> (22.5425, 231.898472)
  line L2981 (22.5425, 231.898472) -> (22.895278, 232.004305)
  line L2982 (39.934444, 235.073472) -> (39.899167, 235.144028)
  line L2983 (39.899167, 235.144028) -> (39.863889, 235.179305)
  line L2984 (31.467778, 228.970417) -> (31.467778, 228.899861)
  line L2985 (38.276389, 295.186805) -> (38.205833, 295.257361)
  line L2986 (4.550833, 222.549861) -> (1.446389, 219.445417)
  line L2987 (1.446389, 218.034306) -> (4.974167, 218.034306)
  line L2988 (23.1775, 287.778472) -> (23.212778, 287.81375)
  line L2989 (21.448889, 287.707917) -> (22.895278, 287.707917)
  line L2990 (23.953611, 229.323194) -> (23.8125, 229.040972)
  line L2991 (40.781111, 261.46125) -> (40.569444, 261.743472)
  line L2992 (23.8125, 229.040972) -> (23.530278, 228.794028)
  line L2993 (17.215556, 290.812361) -> (16.968611, 290.918194)
  line L2994 (9.736667, 231.404583) -> (9.383889, 231.369305)
  line L2995 (22.260278, 230.699028) -> (22.189722, 230.910694)
  line L2996 (22.189722, 230.910694) -> (22.154444, 231.157639)
  line L2997 (22.154444, 231.157639) -> (22.189722, 231.404583)
  line L2998 (24.341667, 253.594305) -> (24.271111, 253.594305)
  line L2999 (36.900556, 272.291528) -> (36.971111, 272.25625)
  line L3000 (36.971111, 272.25625) -> (37.076944, 272.25625)
  line L3001 (36.865278, 272.679583) -> (36.83, 272.57375)
  line L3002 (41.627778, 263.542639) -> (41.733611, 263.542639)
  line L3003 (22.260278, 230.699028) -> (22.330833, 230.557917)
  line L3004 (22.330833, 230.557917) -> (22.471944, 230.416805)
  line L3005 (5.961944, 223.184861) -> (5.856111, 223.325972)
  line L3006 (5.856111, 223.325972) -> (5.856111, 223.467083)
  line L3007 (40.675278, 262.907639) -> (40.781111, 262.590139)
  line L3008 (23.8125, 231.61625) -> (23.671389, 231.792639)
  line L3009 (23.671389, 231.792639) -> (23.495, 231.93375)
  line L3010 (32.102778, 223.149583) -> (32.173333, 223.220139)
  line L3011 (32.173333, 223.220139) -> (32.208611, 223.255417)
  line L3012 (32.208611, 223.255417) -> (32.243889, 223.396528)
  line L3013 (23.283333, 250.384028) -> (23.318611, 250.34875)
  line L3014 (23.318611, 250.34875) -> (23.459722, 250.313472)
  line L3015 (23.283333, 250.66625) -> (23.248056, 250.560417)
  line L3016 (23.248056, 250.560417) -> (23.248056, 250.489861)
  line L3017 (42.262778, 272.362083) -> (42.333333, 272.291528)
  line L3018 (42.333333, 272.291528) -> (42.403889, 272.25625)
  line L3019 (34.536944, 223.255417) -> (34.466389, 223.149583)
  line L3020 (19.120556, 239.765417) -> (19.261667, 239.095139)
  line L3021 (19.261667, 239.095139) -> (19.473333, 238.424861)
  line L3022 (19.473333, 238.424861) -> (19.755556, 237.789861)
  line L3023 (33.196389, 226.85375) -> (34.043056, 226.85375)
  line L3024 (32.843611, 227.135972) -> (32.878889, 227.030139)
  line L3025 (32.878889, 227.030139) -> (32.914167, 226.959583)
  line L3026 (40.886944, 265.130139) -> (41.133889, 265.306528)
  line L3027 (41.133889, 265.306528) -> (41.521944, 265.377083)
  line L3028 (40.146111, 263.260417) -> (40.181389, 263.719028)
  line L3029 (36.794722, 272.503194) -> (36.83, 272.397361)
  line L3030 (36.83, 272.397361) -> (36.900556, 272.291528)
  line L3031 (43.285833, 281.745972) -> (38.346944, 281.745972)
  line L3032 (17.885833, 281.745972) -> (12.946944, 281.745972)
  line L3033 (11.535833, 281.745972) -> (6.596944, 281.745972)
  line L3034 (40.3225, 231.404583) -> (40.216667, 231.863194)
  line L3035 (40.216667, 231.863194) -> (40.005, 232.25125)
  line L3036 (40.3225, 240.470972) -> (40.287222, 240.400417)
  line L3037 (34.043056, 286.402639) -> (33.901944, 286.261528)
  line L3038 (33.901944, 286.261528) -> (33.760833, 286.155694)
  line L3039 (40.181389, 263.719028) -> (40.287222, 264.142361)
  line L3040 (36.83, 272.57375) -> (36.794722, 272.503194)
  line L3041 (36.865278, 272.714861) -> (36.865278, 272.679583)
  line L3042 (34.113611, 223.220139) -> (34.043056, 223.290694)
  line L3043 (16.968611, 290.918194) -> (16.721667, 291.024028)
  line L3044 (38.488056, 249.502083) -> (38.523333, 249.537361)
  line L3045 (26.176111, 224.772361) -> (26.140833, 224.878194)
  line L3046 (22.754167, 230.734305) -> (22.648333, 230.804861)
  line L3047 (23.318611, 230.593194) -> (22.86, 230.699028)
  line L3048 (31.644167, 225.513194) -> (31.644167, 225.58375)
  line L3049 (31.644167, 225.58375) -> (31.608889, 225.689583)
  line L3050 (31.608889, 225.689583) -> (31.538333, 225.724861)
  line L3051 (41.380833, 263.295694) -> (41.416111, 263.401528)
  line L3052 (34.572222, 223.431805) -> (34.572222, 223.36125)
  line L3053 (21.872222, 223.114305) -> (22.225, 223.184861)
  line L3054 (22.225, 223.184861) -> (22.5425, 223.290694)
  line L3055 (31.538333, 225.724861) -> (31.326667, 225.760139)
  line L3056 (31.291389, 225.26625) -> (31.538333, 225.301528)
  line L3057 (23.495, 231.93375) -> (23.353889, 232.004305)
  line L3058 (23.353889, 232.004305) -> (23.1775, 232.004305)
  line L3059 (31.538333, 225.301528) -> (31.573611, 225.336805)
  line L3060 (31.573611, 225.336805) -> (31.608889, 225.372083)
  line L3061 (31.608889, 225.372083) -> (31.644167, 225.513194)
  line L3062 (24.13, 253.453194) -> (23.283333, 250.66625)
  line L3063 (22.895278, 231.61625) -> (22.824722, 231.580972)
  line L3064 (22.824722, 231.580972) -> (22.718889, 231.545694)
  line L3065 (22.718889, 231.545694) -> (22.613056, 231.369305)
  line L3066 (15.804444, 227.382917) -> (16.016111, 227.347639)
  line L3067 (34.184167, 223.149583) -> (34.113611, 223.220139)
  line L3068 (12.453056, 227.347639) -> (12.347222, 227.382917)
  line L3069 (12.594167, 223.431805) -> (12.594167, 227.100694)
  line L3070 (12.311944, 223.114305) -> (12.453056, 223.149583)
  line L3071 (29.421667, 223.184861) -> (29.5275, 223.114305)
  line L3072 (9.913056, 223.255417) -> (9.913056, 223.36125)
  line L3073 (9.913056, 223.36125) -> (9.913056, 223.467083)
  line L3074 (9.489722, 227.312361) -> (9.595556, 227.347639)
  line L3075 (40.287222, 264.142361) -> (40.534167, 264.671528)
  line L3076 (21.448889, 226.712639) -> (21.237222, 226.500972)
  line L3077 (34.043056, 223.396528) -> (34.043056, 223.467083)
  line L3078 (25.153056, 250.313472) -> (25.223611, 250.313472)
  line L3079 (24.906111, 250.842639) -> (25.011944, 250.454583)
  line L3080 (23.777222, 250.842639) -> (24.906111, 250.842639)
  line L3081 (7.584722, 232.498194) -> (7.443611, 232.815694)
  line L3082 (28.151667, 227.17125) -> (28.151667, 227.030139)
  line L3083 (31.855833, 226.85375) -> (31.996944, 226.85375)
  line L3084 (22.648333, 230.804861) -> (22.754167, 230.734305)
  line L3085 (22.754167, 230.734305) -> (22.86, 230.699028)
  line L3086 (22.86, 230.699028) -> (23.318611, 230.593194)
  line L3087 (40.534167, 264.671528) -> (40.886944, 265.130139)
  line L3088 (40.463611, 249.607917) -> (40.428333, 249.537361)
  line L3089 (25.646944, 224.878194) -> (25.611667, 224.737083)
  line L3090 (25.611667, 224.737083) -> (25.611667, 224.63125)
  line L3091 (39.863889, 235.179305) -> (39.6875, 235.214583)
  line L3092 (39.652222, 234.755972) -> (39.758056, 234.755972)
  line L3093 (26.281944, 287.884305) -> (27.375556, 286.014583)
  line L3094 (25.893889, 225.019305) -> (25.752778, 224.984028)
  line L3095 (25.752778, 224.984028) -> (25.646944, 224.878194)
  line L3096 (26.140833, 224.878194) -> (26.105556, 224.94875)
  line L3097 (22.930556, 226.889028) -> (22.683611, 227.100694)
  line L3098 (22.683611, 227.100694) -> (22.401389, 227.277083)
  line L3099 (21.695833, 223.67875) -> (21.484167, 223.749305)
  line L3100 (21.484167, 223.749305) -> (21.201944, 223.99625)
  line L3101 (22.507222, 223.960972) -> (22.401389, 223.819861)
  line L3102 (34.536944, 242.869861) -> (34.360556, 243.540139)
  line L3103 (34.360556, 243.540139) -> (34.113611, 244.210417)
  line L3104 (34.113611, 244.210417) -> (33.831389, 244.845417)
  line L3105 (33.831389, 244.845417) -> (33.478611, 245.445139)
  line L3106 (7.443611, 232.815694) -> (7.337778, 233.168472)
  line L3107 (34.889722, 276.454305) -> (34.783889, 276.489583)
  line L3108 (34.783889, 276.489583) -> (34.713333, 276.489583)
  line L3109 (36.089167, 272.644305) -> (34.995556, 276.242639)
  line L3110 (21.766389, 225.26625) -> (21.801667, 225.125139)
  line L3111 (21.801667, 225.125139) -> (21.872222, 225.054583)
  line L3112 (7.337778, 233.168472) -> (7.3025, 233.52125)
  line L3113 (24.271111, 253.594305) -> (24.200556, 253.559028)
  line L3114 (24.200556, 253.559028) -> (24.165278, 253.52375)
  line L3115 (24.165278, 253.52375) -> (24.13, 253.453194)
  line L3116 (31.996944, 226.85375) -> (32.102778, 226.889028)
  line L3117 (32.102778, 226.889028) -> (32.138056, 226.924305)
  line L3118 (32.138056, 226.924305) -> (32.173333, 226.994861)
  line L3119 (31.291389, 291.270972) -> (31.256111, 291.165139)
  line L3120 (16.016111, 227.347639) -> (16.086667, 227.277083)
  line L3121 (28.469167, 230.769583) -> (27.6225, 230.769583)
  line L3122 (28.716111, 230.557917) -> (28.716111, 230.628472)
  line L3123 (9.913056, 226.112917) -> (9.913056, 223.467083)
  line L3124 (40.428333, 249.537361) -> (40.357778, 249.466805)
  line L3125 (18.908889, 225.724861) -> (18.803056, 225.58375)
  line L3126 (18.803056, 225.58375) -> (18.626667, 225.477917)
  line L3127 (31.256111, 291.165139) -> (31.185556, 291.094583)
  line L3128 (8.748889, 227.100694) -> (8.713611, 226.994861)
  line L3129 (8.713611, 226.994861) -> (8.678333, 226.924305)
  line L3130 (40.393056, 262.060972) -> (40.569444, 261.743472)
  line L3131 (40.886944, 265.130139) -> (40.534167, 264.671528)
  line L3132 (4.974167, 218.034306) -> (9.454444, 222.549861)
  line L3133 (43.991389, 218.986806) -> (43.991389, 222.549861)
  line L3134 (42.650833, 222.549861) -> (38.135278, 218.034306)
  line L3135 (38.135278, 218.034306) -> (43.074167, 218.034306)
  line L3136 (43.074167, 218.034306) -> (43.991389, 218.986806)
  line L3137 (33.760833, 286.155694) -> (33.443333, 286.085139)
  line L3138 (35.806944, 289.507083) -> (35.806944, 289.648194)
  line L3139 (13.335, 257.898194) -> (13.476111, 257.615972)
  line L3140 (22.613056, 231.369305) -> (22.5425, 231.157639)
  line L3141 (22.5425, 231.157639) -> (22.577778, 230.98125)
  line L3142 (22.577778, 230.98125) -> (22.648333, 230.804861)
  line L3143 (31.291389, 291.341528) -> (31.291389, 291.270972)
  line L3144 (28.469167, 253.594305) -> (28.398611, 253.594305)
  line L3145 (28.398611, 253.594305) -> (28.328056, 253.559028)
  line L3146 (23.883056, 231.228194) -> (23.847778, 231.439861)
  line L3147 (23.847778, 231.439861) -> (23.8125, 231.61625)
  line L3148 (31.185556, 291.094583) -> (31.079722, 291.059305)
  line L3149 (8.501944, 223.643472) -> (8.5725, 223.643472)
  line L3150 (8.5725, 223.643472) -> (8.713611, 223.537639)
  line L3151 (33.9725, 241.14125) -> (33.937222, 241.811528)
  line L3152 (33.937222, 241.811528) -> (33.831389, 242.446528)
  line L3153 (33.831389, 242.446528) -> (33.690278, 243.116805)
  line L3154 (33.690278, 243.116805) -> (33.478611, 243.716528)
  line L3155 (33.478611, 243.716528) -> (33.231667, 244.31625)
  line L3156 (33.231667, 244.31625) -> (32.914167, 244.880694)
  line L3157 (32.914167, 244.880694) -> (32.526111, 245.445139)
  line L3158 (32.526111, 245.445139) -> (32.102778, 245.939028)
  line L3159 (32.102778, 245.939028) -> (31.644167, 246.397639)
  line L3160 (31.644167, 246.397639) -> (31.150278, 246.820972)
  line L3161 (31.150278, 246.820972) -> (30.585833, 247.209028)
  line L3162 (30.585833, 247.209028) -> (30.021389, 247.526528)
  line L3163 (30.021389, 247.526528) -> (29.421667, 247.773472)
  line L3164 (29.421667, 247.773472) -> (28.786667, 247.985139)
  line L3165 (28.786667, 247.985139) -> (28.151667, 248.161528)
  line L3166 (28.151667, 248.161528) -> (27.516667, 248.232083)
  line L3167 (27.516667, 248.232083) -> (26.846389, 248.267361)
  line L3168 (26.846389, 248.267361) -> (26.211389, 248.232083)
  line L3169 (26.211389, 248.232083) -> (25.541111, 248.161528)
  line L3170 (25.541111, 248.161528) -> (24.906111, 247.985139)
  line L3171 (24.906111, 247.985139) -> (24.271111, 247.773472)
  line L3172 (24.271111, 247.773472) -> (23.671389, 247.526528)
  line L3173 (23.671389, 247.526528) -> (23.106944, 247.209028)
  line L3174 (23.106944, 247.209028) -> (22.577778, 246.820972)
  line L3175 (22.577778, 246.820972) -> (22.048611, 246.397639)
  line L3176 (22.048611, 246.397639) -> (21.59, 245.939028)
  line L3177 (21.59, 245.939028) -> (21.166667, 245.445139)
  line L3178 (21.166667, 245.445139) -> (20.813889, 244.880694)
  line L3179 (20.813889, 244.880694) -> (20.496389, 244.31625)